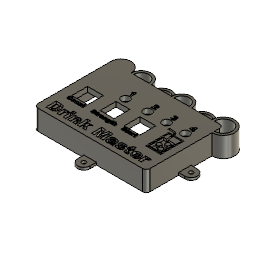
UIHolder (Autodesk Fusion 360 design; units mm, degrees)
part number: 2026-05-20-16-52-47-232
Autodesk Fusion 360 part; units mm, degrees
note: some values were not read from the file. Set by a fixed rule: which sketch regions a step uses.
sketch "Sketch1" plane through (0, 0, 0) normal (0, 0, 1) x (1, 0, 0)
  line L0 (0, 0) -> (0, 57)
  line L1 (0, 0) -> (85, 0)
  line L2 (0, 57) -> (85, 57)
  line L3 (85, 57) -> (85, 0)
  line L4 (-2, 59) -> (87, 59)
  line L5 (87, 59) -> (87, -2)
  line L6 (87, -2) -> (-2, -2)
  line L7 (-2, -2) -> (-2, 59)
  circle A0 centre (6, 59) radius 6
  circle A1 centre (6, 59) radius 8
  line L8 (0, 59) -> (0, 57)
  line L9 (12, 59) -> (12, 57)
  circle A2 centre (77, 39) radius 3.25
  circle A3 centre (62, 39) radius 3.25
  circle A4 centre (47, 39) radius 3.25
  circle A5 centre (29.5, 39) radius 3.25
  line L10 (47.5, 32.5) -> (60, 32.5)
  line L11 (60, 32.5) -> (60, 20)
  line L12 (60, 20) -> (47.5, 20)
  line L13 (47.5, 20) -> (47.5, 32.5)
  line L14 (6, 20) -> (18.5, 20)
  line L15 (18.5, 20) -> (18.5, 32.5)
  line L16 (18.5, 32.5) -> (6, 32.5)
  line L17 (6, 32.5) -> (6, 20)
  line L18 (27.5, 33.5) -> (38.5, 33.5)
  line L19 (38.5, 33.5) -> (38.5, 21)
  line L20 (38.5, 21) -> (27.5, 21)
  line L21 (27.5, 21) -> (27.5, 33.5)
  circle A6 centre (22, 59) radius 8
  circle A7 centre (22, 59) radius 6
  circle A8 centre (38, 59) radius 8
  circle A9 centre (38, 59) radius 6
  circle A10 centre (54, 59) radius 8
  circle A11 centre (54, 59) radius 6
  circle A12 centre (70, 59) radius 8
  circle A13 centre (70, 59) radius 6
  circle A14 centre (87, 59) radius 9
  circle A15 centre (87, 59) radius 7
  circle A16 centre (-7, 28.5) radius 1.65
  circle A17 centre (42.5, -7) radius 1.65
  circle A18 centre (92, 28.5) radius 1.65
  line L22 (-2, 23.5) -> (-12, 23.5)
  line L23 (-12, 23.5) -> (-12, 33.5)
  line L24 (-12, 33.5) -> (-2, 33.5)
  line L25 (-2, 33.5) -> (-2, 23.5)
  line L26 (-2, 23.5) -> (-12, 33.5) construction
  line L27 (-12, 23.5) -> (-2, 33.5) construction
  line L28 (47.5, -2) -> (37.5, -2)
  line L29 (37.5, -2) -> (37.5, -12)
  line L30 (37.5, -12) -> (47.5, -12)
  line L31 (47.5, -12) -> (47.5, -2)
  line L32 (47.5, -2) -> (37.5, -12) construction
  line L33 (37.5, -2) -> (47.5, -12) construction
  line L34 (87, 23.5) -> (97, 23.5)
  line L35 (97, 23.5) -> (97, 33.5)
  line L36 (97, 33.5) -> (87, 33.5)
  line L37 (87, 33.5) -> (87, 23.5)
  line L38 (87, 23.5) -> (97, 33.5) construction
  line L39 (97, 23.5) -> (87, 33.5) construction
  point P0 (-7, 28.5)
  point P1 (42.5, -7)
  point P2 (92, 28.5)
  dimension "d1" = 57
  dimension "d2" = 85
  dimension "d3" = 85
  dimension "d4" = 2
  dimension "d5" = 2
  dimension "d6" = 2
  dimension "d7" = 2
  dimension "d8" = 12
  dimension "d9" = 8
  dimension "d12" = 6.5
  dimension "d13" = 8
  dimension "d15" = 6.5
  dimension "d17" = 15
  dimension "d18" = 6.5
  dimension "d20" = 15
  dimension "d21" = 6.5
  dimension "d22" = 18
  dimension "d23" = 18
  dimension "d24" = 18
  dimension "d25" = 18
  dimension "d26" = 17.5
  dimension "d27" = 12.5
  dimension "d28" = 12.5
  dimension "d29" = 25
  dimension "d30" = 20
  dimension "d31" = 12.5
  dimension "d32" = 12.5
  dimension "d33" = 20
  dimension "d34" = 6
  dimension "d35" = 12.5
  dimension "d36" = 11
  dimension "d37" = 9
  dimension "d38" = 21
  dimension "d42" = 16
  dimension "d43" = 12
  dimension "d44" = 16
  dimension "d45" = 12
  dimension "d46" = 16
  dimension "d47" = 12
  dimension "d48" = 16
  dimension "d49" = 12
  dimension "d50" = 14
  dimension "d75" = 3.3
  dimension "d76" = 3.3
  dimension "d77" = 3.3
  dimension "d78" = 30.5
  dimension "d79" = 30.5
  dimension "d80" = 44.5
  dimension "d81" = 5
  dimension "d82" = 5
  dimension "d83" = 5
  dimension "d84" = 10
  dimension "d85" = 10
  dimension "d86" = 10
  dimension "d87" = 10
  dimension "d88" = 10
  dimension "d89" = 10
  constraint coincident L0.start L1.start
  constraint vertical L0
  constraint perpendicular L0 L1
  constraint perpendicular L0 L2
  constraint horizontal L4
  constraint vertical L5
  constraint horizontal L6
  constraint vertical L7
  constraint coincident L4 A0.centre
  constraint concentric A0 A1
  constraint coincident L4.start A1
  constraint coincident A0 L8.start
  constraint coincident L4 L8.start
  constraint coincident L4 L9.start
  constraint coincident A0 L9.start
  constraint coincident L2 L9.end
  constraint perpendicular L2 L9
  constraint horizontal L10
  constraint vertical L11
  constraint horizontal L12
  constraint vertical L13
  constraint horizontal L14
  constraint vertical L15
  constraint horizontal L16
  constraint vertical L17
  constraint horizontal L18
  constraint vertical L19
  constraint horizontal L20
  constraint vertical L21
  constraint coincident L4 A6.centre
  constraint tangent A1 A6
  constraint concentric A6 A7
  constraint coincident L4 A8.centre
  constraint tangent A6 A8
  constraint concentric A8 A9
  constraint coincident L4 A10.centre
  constraint tangent A8 A10
  constraint concentric A10 A11
  constraint coincident L4 A12.centre
  constraint tangent A10 A12
  constraint concentric A12 A13
  constraint coincident L4.end L5.start
  constraint tangent A12 A14
  constraint concentric A14 A15
  constraint horizontal L22
  constraint perpendicular L22 L23
  constraint parallel L22 L24
  constraint parallel L23 L25
  constraint coincident L26 P0
  constraint coincident L27 P0
  constraint coincident P0 A16.centre
  constraint horizontal L28
  constraint perpendicular L28 L29
  constraint parallel L28 L30
  constraint parallel L29 L31
  constraint coincident L32 P1
  constraint coincident L33 P1
  constraint coincident P1 A17.centre
  constraint horizontal L34
  constraint perpendicular L34 L35
  constraint parallel L34 L36
  constraint parallel L35 L37
  constraint coincident L38 P2
  constraint coincident L39 P2
  constraint coincident P2 A18.centre
  measures "d1" distance of L0.start L0.end
  measures "d2" distance of L0.start L1.end
  measures "d3" distance of L0.end L2.end
  measures "d4" distance of L2 L4
  measures "d5" distance of L0 L7
  measures "d6" distance of L1 L6
  measures "d7" distance of L3 L5
  measures "d8" diameter of A0
  measures "d9" distance of L4.start A0.centre
  measures "d12" diameter of A2
  measures "d13" distance of L3 A2.centre
  measures "d15" diameter of A3
  measures "d17" distance of A2.centre A3.centre
  measures "d18" diameter of A4
  measures "d20" distance of A3.centre A4.centre
  measures "d21" diameter of A5
  measures "d22" distance of L2 A5.centre
  measures "d23" distance of L2 A4.centre
  measures "d24" distance of L2 A3.centre
  measures "d25" distance of L2 A2.centre
  measures "d26" distance of A4.centre A5.centre
  measures "d27" distance of L10.start L10.end
  measures "d28" distance of L10.start L12.end
  measures "d29" distance of L3 L11
  measures "d30" distance of L1 L12
  measures "d31" distance of L15.end L16.end
  measures "d32" distance of L14.end L15.end
  measures "d33" distance of L1 L14
  measures "d34" distance of L0 L17
  measures "d35" distance of L18.start L20.end
  measures "d36" distance of L18.start L18.end
  measures "d37" distance of L13 L19
  measures "d38" distance of L1 L20
  measures "d42" diameter of A6
  measures "d43" diameter of A7
  measures "d44" diameter of A8
  measures "d45" diameter of A9
  measures "d46" diameter of A10
  measures "d47" diameter of A11
  measures "d48" diameter of A12
  measures "d49" diameter of A13
  measures "d50" diameter of A15
  measures "d75" diameter of A16
  measures "d76" diameter of A17
  measures "d77" diameter of A18
  measures "d78" vertical distance of L4.start P0
  measures "d79" vertical distance of L4.end P2
  measures "d80" horizontal distance of L5.end P1
  measures "d81" distance of L6 P1
  measures "d82" distance of L7 P0
  measures "d83" distance of L5 P2
  measures "d84" distance of L22.end L23.end
  measures "d85" distance of L22.start L22.end
  measures "d86" distance of L29.end L30.end
  measures "d87" distance of L28.start L30.end
  measures "d88" distance of L34.end L35.end
  measures "d89" distance of L35.end L36.end
extrude "Extrude4" add sketch "Sketch1" along normal blind 2 contours L7 L22 L23 L24 L25 | L5 L34 L35 L36 L37 | L6 L28 L29 L30 L31 makes body 1 at (-7.0411, 24.6182, 0) makes body 2 at (42.5411, -3.1182, 0) makes body 3 at (91.9589, 24.6182, 0)
fillet "Fillet4" radius 5 6 edges at (-12, 23.5, 1) (-12, 33.5, 1) (37.5, -12, 1) (47.5, -12, 1) (97, 23.5, 1) (97, 33.5, 1) on bodies 1 2 3
extrude "Extrude1" add sketch "Sketch1" along normal blind 12 contours L0 L1 L3 L5 L6 L7 A1 A14 L25 L28 L37 | L0 L4 A1 L8 | L4 A0 A1 | L2 A1 A6 | L2 L4 A1 L9 | L3 L5 A14 A15 | L4 A6 A7 | L2 L4 A6 A7 | L2 L3 L4 L5 A15 | L2 L4 A14 A15 | L2 A12 A14 | L4 L5 A14 A15 | L2 L4 A7 | L2 L4 A6 A7 | L4 A8 A9 | L2 A6 A8 | L2 L4 A8 A9 | L2 L4 A12 A13 | L4 A12 A13 | L2 L4 A9 | L2 L4 A8 A9 | L4 A10 A11 | L2 A8 A10 | L2 L4 A10 A11 | L2 L4 A13 | L2 L4 A12 A13 | L2 A10 A12 | L2 L4 A10 A11 | L2 L4 A11 bodies 1 2 3
extrude "Extrude2" add sketch "Sketch1" along normal blind 4 from surface at 12 contours L0 L1 L3 L5 L6 L7 A1 A14 L25 L28 L37 | L0 L1 L2 L3 A1 A6 A8 A10 A12 A14 | L0 L4 A1 L8 | L0 L2 A0 A1 | L2 A0 L8 | L4 A0 A1 | L2 A1 A6 | L2 L4 A1 L9 | L2 L3 A14 A15 | L3 L5 A14 A15 | L2 L4 A0 | L2 A0 | L4 A0 | L4 A6 A7 | L2 L4 A6 A7 | L2 A0 L9 | L2 A6 A7 | L2 L3 A15 | L2 L3 L4 L5 A15 | L2 L4 A14 A15 | L2 A12 A14 | L4 L5 A14 A15 | L2 L4 A7 | L2 L4 A6 A7 | L2 A6 A8 | L2 L4 A8 A9 | L2 A7 | L2 A12 A13 | L2 L4 A12 A13 | L2 L4 A9 | L2 L4 A8 A9 | L4 A10 A11 | L2 A8 A10 | L2 L4 A10 A11 | L2 A8 A9 | L2 A13 | L2 L4 A13 | L2 L4 A12 A13 | L2 A10 A12 | L2 L4 A10 A11 | L2 A9 | L2 L4 A11 | L2 A10 A11 | L2 A11 bodies 1
fillet "Fillet3" radius 3 7 edges at (85, 57, 6) (87, 59, 8) (87, -2, 8) (85, 0, 6) (-2, -2, 8) (12, 57, 6) (0, 0, 6) on bodies 1
sketch "Sketch2" plane through (0, 0, 16) normal (0, 0, 1) x (-1, 0, 0)
  line L0 (-60, -32.5) -> (-60, -20)
  line L1 (-60, -20) -> (-47.5, -20)
  line L2 (-47.5, -20) -> (-47.5, -32.5)
  line L3 (-47.5, -32.5) -> (-60, -32.5)
  circle A0 centre (-47, -39) radius 3.25
  line L4 (-18.5, -20) -> (-6, -20)
  line L5 (-6, -20) -> (-6, -32.5)
  line L6 (-6, -32.5) -> (-18.5, -32.5)
  line L7 (-18.5, -32.5) -> (-18.5, -20)
  line L8 (-60, -59) -> (-48, -59)
  arc A1 (-60, -59) -> (-48, -59) centre (-54, -59) ccw
  circle A2 centre (-29.5, -39) radius 3.25
  circle A3 centre (-77, -39) radius 3.25
  arc A4 (-87, -56) -> (-84, -59) centre (-84, -56) ccw
  line L9 (-84, -59) -> (-80, -59)
  arc A5 (-87, -52) -> (-80, -59) centre (-87, -59) ccw
  line L10 (-87, -52) -> (-87, -56)
  line L11 (-38.5, -33.5) -> (-38.5, -21)
  line L12 (-38.5, -21) -> (-27.5, -21)
  line L13 (-27.5, -21) -> (-27.5, -33.5)
  line L14 (-27.5, -33.5) -> (-38.5, -33.5)
  line L15 (-28, -59) -> (-16, -59)
  arc A6 (-28, -59) -> (-16, -59) centre (-22, -59) ccw
  circle A7 centre (-62, -39) radius 3.25
  arc A8 (2, -1) -> (-1, 2) centre (-1, -1) ccw
  line L16 (-1, 2) -> (-84, 2)
  arc A9 (-84, 2) -> (-87, -1) centre (-84, -1) ccw
  line L17 (-87, -1) -> (-87, -50)
  arc A10 (-87, -50) -> (-78, -59) centre (-87, -59) ccw
  line L18 (-78, -59) -> (-62, -59)
  arc A11 (-62, -59) -> (-46, -59) centre (-54, -59) ccw
  line L19 (-46, -59) -> (-30, -59)
  arc A12 (-30, -59) -> (-14, -59) centre (-22, -59) ccw
  arc A13 (-14, -59) -> (2, -59) centre (-6, -59) ccw
  line L20 (2, -59) -> (2, -1)
  line L21 (0, 5) -> (-85, 5) construction
  line L22 (-85, 5) -> (-85, -10) construction
  line L23 (-85, -10) -> (0, -10) construction
  line L24 (0, -10) -> (0, 5) construction
  line L25 (-80.7167, -33.0536) -> (-73.974, -33.0536)
  line L26 (-73.974, -33.0536) -> (-73.8798, -33.7934)
  spline S0 degree 3 poles (-73.8798, -33.7934) (-73.8174, -34.4845) (-73.2798, -35.8297) (-71.6997, -35.9736) knots 0 0 0 0 1 1 1 1
  spline S1 degree 3 poles (-71.6997, -35.9736) (-70.1704, -36.1122) (-67.2864, -36.2477) (-67.1637, -36.254) knots 0 0 0 0 1 1 1 1
  line L27 (-67.1637, -36.254) -> (-67.1118, -35.1386)
  spline S2 degree 3 poles (-67.1118, -35.1386) (-67.1414, -35.1375) (-70.0942, -34.9978) (-71.5991, -34.8613) knots 0 0 0 0 1 1 1 1
  spline S3 degree 3 poles (-71.5991, -34.8613) (-72.6236, -34.7681) (-72.7569, -33.7987) (-72.7707, -33.6728) knots 0 0 0 0 1 1 1 1
  line L28 (-72.7707, -33.6728) -> (-72.849, -33.0536)
  line L29 (-72.849, -33.0536) -> (-70.5768, -33.0536)
  line L30 (-70.5768, -33.0536) -> (-69.7396, -33.0536)
  line L31 (-69.7396, -33.0536) -> (-69.7396, -32.2165)
  line L32 (-69.7396, -32.2165) -> (-69.7396, -15.6684)
  line L33 (-69.7396, -15.6684) -> (-69.7396, -14.8313)
  line L34 (-69.7396, -14.8313) -> (-70.5768, -14.8313)
  line L35 (-70.5768, -14.8313) -> (-80.7177, -14.8313)
  line L36 (-80.7177, -14.8313) -> (-81.5549, -14.8313)
  line L37 (-81.5549, -14.8313) -> (-81.5549, -15.6684)
  line L38 (-81.5549, -15.6684) -> (-81.5549, -32.2165)
  line L39 (-81.5549, -32.2165) -> (-81.5549, -33.0536)
  line L40 (-81.5549, -33.0536) -> (-80.7167, -33.0536)
  line L41 (-80.7167, -15.6684) -> (-70.5768, -15.6684)
  line L42 (-70.5768, -15.6684) -> (-70.5768, -32.2165)
  line L43 (-70.5768, -32.2165) -> (-72.9549, -32.2165)
  line L44 (-72.9549, -32.2165) -> (-73.5316, -27.6583)
  line L45 (-73.5316, -27.6583) -> (-71.1356, -27.6583)
  line L46 (-71.1356, -27.6583) -> (-71.1356, -16.2272)
  line L47 (-71.1356, -16.2272) -> (-80.1589, -16.2272)
  line L48 (-80.1589, -16.2272) -> (-80.1589, -27.6572)
  line L49 (-80.1589, -27.6572) -> (-74.6577, -27.6572)
  line L50 (-74.6577, -27.6572) -> (-74.0799, -32.2165)
  line L51 (-74.0799, -32.2165) -> (-80.7167, -32.2165)
  line L52 (-80.7167, -32.2165) -> (-80.7167, -15.6684)
  spline S4 degree 3 poles (-75.2059, -22.4015) (-75.498, -22.2967) (-75.6504, -21.975) (-75.5467, -21.6829) knots 0 0 0 0 1 1 1 1
  line L53 (-75.5467, -21.6829) -> (-74.9085, -19.8943)
  spline S5 degree 3 poles (-74.9085, -19.8943) (-74.8038, -19.6022) (-74.482, -19.4488) (-74.1899, -19.5535) knots 0 0 0 0 1 1 1 1
  line L54 (-74.1899, -19.5535) -> (-72.4013, -20.1917)
  spline S6 degree 3 poles (-72.4013, -20.1917) (-72.1082, -20.2965) (-71.9558, -20.6172) (-72.0606, -20.9103) knots 0 0 0 0 1 1 1 1
  line L55 (-72.0606, -20.9103) -> (-72.6977, -22.6989)
  spline S7 degree 3 poles (-72.6977, -22.6989) (-72.8025, -22.991) (-73.1242, -23.1434) (-73.4163, -23.0397) knots 0 0 0 0 1 1 1 1
  line L56 (-73.4163, -23.0397) -> (-75.2059, -22.4015)
  line L57 (-79.216, -25.0854) -> (-78.5778, -23.2969)
  spline S8 degree 3 poles (-78.5778, -23.2969) (-78.473, -23.0048) (-78.1513, -22.8513) (-77.8592, -22.9571) knots 0 0 0 0 1 1 1 1
  line L58 (-77.8592, -22.9571) -> (-76.0706, -23.5943)
  spline S9 degree 3 poles (-76.0706, -23.5943) (-75.7785, -23.699) (-75.625, -24.0197) (-75.7309, -24.3129) knots 0 0 0 0 1 1 1 1
  line L59 (-75.7309, -24.3129) -> (-76.368, -26.1014)
  spline S10 degree 3 poles (-76.368, -26.1014) (-76.4738, -26.3946) (-76.7934, -26.547) (-77.0866, -26.4422) knots 0 0 0 0 1 1 1 1
  line L60 (-77.0866, -26.4422) -> (-78.8752, -25.8051)
  spline S11 degree 3 poles (-78.8752, -25.8051) (-79.1662, -25.6993) (-79.3197, -25.3775) (-79.216, -25.0854) knots 0 0 0 0 1 1 1 1
  spline S12 degree 3 poles (-79.4869, -18.4) (-79.5948, -18.11) (-79.4456, -17.7851) (-79.1546, -17.6771) knots 0 0 0 0 1 1 1 1
  line L61 (-79.1546, -17.6771) -> (-77.3723, -17.0188)
  spline S13 degree 3 poles (-77.3723, -17.0188) (-77.0824, -16.9098) (-76.7585, -17.0601) (-76.6506, -17.3501) knots 0 0 0 0 1 1 1 1
  line L62 (-76.6506, -17.3501) -> (-75.9912, -19.1323)
  spline S14 degree 3 poles (-75.9912, -19.1323) (-75.8833, -19.4234) (-76.0325, -19.7462) (-76.3235, -19.8552) knots 0 0 0 0 1 1 1 1
  line L63 (-76.3235, -19.8552) -> (-78.1058, -20.5134)
  spline S15 degree 3 poles (-78.1058, -20.5134) (-78.3957, -20.6214) (-78.7196, -20.4722) (-78.8275, -20.1811) knots 0 0 0 0 1 1 1 1
  line L64 (-78.8275, -20.1811) -> (-79.4869, -18.4)
  line L65 (-23.8535, -40.2294) -> (-33.8535, -40.2294) construction
  line L66 (-33.8535, -40.2294) -> (-33.8535, -47.2294) construction
  line L67 (-33.8535, -47.2294) -> (-23.8535, -47.2294) construction
  line L68 (-23.8535, -47.2294) -> (-23.8535, -40.2294) construction
  line L69 (-42.0223, -40.2294) -> (-52.0223, -40.2294) construction
  line L70 (-52.0223, -40.2294) -> (-52.0223, -47.2294) construction
  line L71 (-52.0223, -47.2294) -> (-42.0223, -47.2294) construction
  line L72 (-42.0223, -47.2294) -> (-42.0223, -40.2294) construction
  line L73 (-57.0223, -40.2294) -> (-67.0223, -40.2294) construction
  line L74 (-67.0223, -40.2294) -> (-67.0223, -47.2294) construction
  line L75 (-67.0223, -47.2294) -> (-57.0223, -47.2294) construction
  line L76 (-57.0223, -47.2294) -> (-57.0223, -40.2294) construction
  line L77 (-72.0223, -40.2294) -> (-82.0223, -40.2294) construction
  line L78 (-82.0223, -40.2294) -> (-82.0223, -47.2294) construction
  line L79 (-82.0223, -47.2294) -> (-72.0223, -47.2294) construction
  line L80 (-72.0223, -47.2294) -> (-72.0223, -40.2294) construction
  line L81 (-6.9491, -12.274) -> (-16.9491, -12.274) construction
  line L82 (-16.9491, -12.274) -> (-16.9491, -19.274) construction
  line L83 (-16.9491, -19.274) -> (-6.9491, -19.274) construction
  line L84 (-6.9491, -19.274) -> (-6.9491, -12.274) construction
  line L85 (-28.9491, -12.274) -> (-38.9491, -12.274) construction
  line L86 (-38.9491, -12.274) -> (-38.9491, -19.274) construction
  line L87 (-38.9491, -19.274) -> (-28.9491, -19.274) construction
  line L88 (-28.9491, -19.274) -> (-28.9491, -12.274) construction
  line L89 (-48.8026, -12.3696) -> (-58.8026, -12.3696) construction
  line L90 (-58.8026, -12.3696) -> (-58.8026, -19.3696) construction
  line L91 (-58.8026, -19.3696) -> (-48.8026, -19.3696) construction
  line L92 (-48.8026, -19.3696) -> (-48.8026, -12.3696) construction
  dimension "d57" = 8
  dimension "d59" = 4
  dimension "d60" = 0
  dimension "d61" = 4
  dimension "d62" = 0
  dimension "d63" = 4
  dimension "d64" = 0
  dimension "d65" = 4
  dimension "d66" = 0
  dimension "d67" = 3
  dimension "d69" = 3
  dimension "d71" = 3
  text T0 "Drink Master" font "Arial Black" height 8 align centre top in box 85 x 15 at (0, 5) x (-1, 0) y (0, -1) spacing 1
  text T1 "1" font "Arial Black" height 4 align centre top in box 10 x 7 at (-23.8535, -40.2294) x (-1, 0) y (0, -1) spacing 1
  text T2 "2" font "Arial Black" height 4 align centre top in box 10 x 7 at (-42.0223, -40.2294) x (-1, 0) y (0, -1) spacing 1
  text T3 "3" font "Arial Black" height 4 align centre top in box 10 x 7 at (-57.0223, -40.2294) x (-1, 0) y (0, -1) spacing 1
  text T4 "4" font "Arial Black" height 4 align centre top in box 10 x 7 at (-72.0223, -40.2294) x (-1, 0) y (0, -1) spacing 1
  text T5 "Count" font "Arial Black" height 3 align centre top in box 10 x 7 at (-6.9491, -12.274) x (-1, 0) y (0, -1) spacing 1
  text T6 "Strength" font "Arial Black" height 3 align centre top in box 10 x 7 at (-28.9491, -12.274) x (-1, 0) y (0, -1) spacing 1
  text T7 "Start" font "Arial Black" height 3 align centre top in box 10 x 7 at (-48.8026, -12.3696) x (-1, 0) y (0, -1) spacing 1
extrude "Extrude3" cut sketch "Sketch2" sketch "Sketch2" against normal blind 2 contours L25 L26 S0 S1 L27 S2 S3 L28 L29 L30 L31 L32 L33 L34 L35 L36 L37 L38 L39 L40 of sketch 2 text T2 T1 T3 T4 T0 T7 T6 T5 bodies 1
equation "d58 = 'Drink Master'"
equation "d60 = '1'"
equation "d62 = '2'"
equation "d64 = '3'"
equation "d66 = '4'"
equation "d68 = 'Count'"
equation "d70 = 'Strength'"
equation "d72 = 'Start'"
